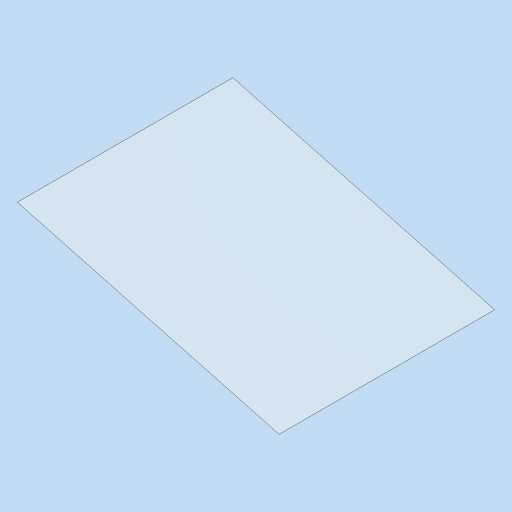
# Autodesk Inventor part: 부품3
Saved by Autodesk Inventor 2024.1 (Build 281209000, 209)
## iProperties
Created: 2024-01-18
Part Number: 부품3
Material: 물
Document SubType Name: Modeling
Designer: likek
Density: 0.9983 g/cm^3
Appearance: 트로피컬 블루
Author: likek
Autodesk Inventor part; units mm, degrees
ref_plane "YZ Plane" through (0, 0, 0) normal (1, 0, 0) x (0, 1, 0)
ref_plane "XZ Plane" through (0, 0, 0) normal (0, 1, 0) x (-1, 0, 0)
ref_plane "XY Plane" through (0, 0, 0) normal (0, 0, 1) x (1, 0, 0)
sketch "스케치1" plane through (0, 0, 0) normal (0, 0, 1) x (1, 0, 0)
  line L0 (0, 0) -> (0, 0.5)
  line L1 (0, 0.5) -> (-850, 228.2568)
  line L2 (-850, 228.2568) -> (-850, 227.7568)
  line L3 (-850, 227.7568) -> (0, 0)
  line L4 (-16.0542, 0) -> (7.8614, 0)
  point P0 (0, 0.25)
  dimension "d0" = 15
  dimension "d1" = 0.5
  dimension "d2" = 850
  constraints: 10 end point, 2 parallel, 1 horizontal, 1 midpoint, 1 vertical
  measures "d0" angle of L3 L4
  measures "d1" distance of L1.end L2.end
  measures "d2" distance from line of point (0, 0.25) L2
extrude "돌출1" add sketch "스케치1" against normal blind 700
